Traktorstift_v2 (Autodesk Fusion 360 design; units mm, degrees)
Autodesk Fusion 360 part; units mm, degrees
cylinder "Grundkörper Zylinder1" add diameter 13.85 height 105 placed x (1, 0, 0) y (0, 0, -1) z (0, 1, 0) at (0, 0, 0)
cylinder "Grundkörper Zylinder2" add diameter 20 height 3 placed x (1, 0, 0) y (0, 0, -1) z (0, 1, 0) at (0, 105, 0)
chamfer "Fase1" distance 0.5 distance2 10 1 edges at (-6.4564, 105, 2.5042) measured on face at (8.912, 105, 0.8408)
sketch "Skizze3" plane through (0, 0, 0) normal (1, 0, 0) x (0, 0, -1)
  line L0 (0, 109) -> (-14.5, 109)
  line L1 (-22.5, 117) -> (-22.5, 129)
  line L2 (-17.5, 134) -> (17.5, 134)
  line L3 (22.5, 129) -> (22.5, 117)
  line L4 (14.5, 109) -> (0, 109)
  arc A0 (-17.5, 134) -> (-22.5, 129) centre (-17.5, 129) ccw
  arc A1 (-22.5, 117) -> (-14.5, 109) centre (-14.5, 117) ccw
  arc A2 (14.5, 109) -> (22.5, 117) centre (14.5, 117) ccw
  arc A3 (22.5, 129) -> (17.5, 134) centre (17.5, 129) ccw
  point P0 (-22.5, 109)
  point P1 (-22.5, 134)
  point P2 (22.5, 134)
  dimension "d7" = 22.5
  dimension "d8" = 25
  dimension "d9" = 45
  dimension "d10" = 5
  dimension "d11" = 8
  dimension "d12" = 8
  dimension "d13" = 5
  constraint horizontal L0
  constraint perpendicular L0 L1
  constraint perpendicular L1 L2
  constraint perpendicular L0 L3
  constraint perpendicular L3 L4
  constraint coincident P1 L1
  constraint coincident P1 L2
  constraint tangent L1 A0
  constraint tangent L2 A0
  constraint coincident P0 L1
  constraint coincident P0 L0
  constraint tangent L1 A1
  constraint tangent L0 A1
  constraint tangent L3 A2
  constraint tangent L4 A2
  constraint coincident P2 L2
  constraint coincident P2 L3
  constraint tangent L2 A3
  constraint tangent L3 A3
  measures "d7" distance of L0.start P0
  measures "d8" distance of P0 P1
  measures "d9" distance of P1 P2
  measures "d10" radius of A0
  measures "d11" radius of A1
  measures "d12" radius of A2
  measures "d13" radius of A3
pipe "Leitung1" add diameter 7 path "Skizze3" along L2 A3 L3 A2 L4 L0 A1 L1 A0
chamfer "Fase2" distance 2 distance2 7 1 edges at (-6.4564, 0, -2.5042) measured on face at (2.4551, 0, -1.9578)
